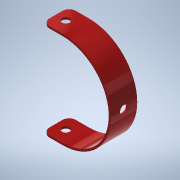
# Autodesk Inventor part: Apoio_Tubo
Saved by Autodesk Inventor 2022 (Build 260153000, 153)
## iProperties
Created: 2016-03-04
Part Number: Apoio_Tubo
Material: Genérico
Document SubType Name: Modeling
Designer: Everton
Density: 1 g/cm^3
Appearance: Padrão
Author: Everton
Autodesk Inventor part; units mm, degrees
ref_plane "YZ Plane" through (0, 0, 0) normal (1, 0, 0) x (0, 1, 0)
ref_plane "XZ Plane" through (0, 0, 0) normal (0, 1, 0) x (-1, 0, 0)
ref_plane "XY Plane" through (0, 0, 0) normal (0, 0, 1) x (1, 0, 0)
sketch "Sketch1" plane through (0, 0, 0) normal (0, 1, 0) x (-1, 0, 0)
  arc A0 (10.8783, 63.6799) -> (10.8783, -82.6701) centre (10.8783, -9.4951) ccw
  line L0 (10.8783, 63.6799) -> (40.8783, 63.6799)
  line L1 (40.8783, -82.6701) -> (10.8783, -82.6701)
  line L2 (40.8783, -79.4951) -> (10.8783, -79.4951)
  arc A1 (10.8783, 60.5049) -> (10.8783, -79.4951) centre (10.8783, -9.4951) ccw
  line L3 (10.8783, 60.5049) -> (40.8783, 60.5049)
  line L4 (40.8783, 63.6799) -> (40.8783, 60.5049)
  line L5 (40.8783, -79.4951) -> (40.8783, -82.6701)
  line L6 (25.8783, -82.6701) -> (25.8783, -9.4951)
  line L7 (25.8783, -9.4951) -> (10.8783, -9.4951)
  dimension "d1" = 30
  dimension "d2" = 3.175
  dimension "d15" = 70
  constraints: 16 end point, 4 point on circle, 2 centre point, 2 vertical, 1 collinear, 1 horizontal, 1 midpoint, 1 perpendicular, 2 other
  measures "d1" distance of L0.start L0.end
  measures "d2" radial gap between concentric circles of A0 A1
  measures "d15" radius of A1
extrude "Extrusion1" add sketch "Sketch1" along normal blind 40
sketch "Sketch2" plane through (-40.8783, 0, 63.6799) normal (0, 0, 1) x (1, 0, 0)
  line L0 (29.9701, 0) -> (0, 40)
  line L1 (0, 40) -> (30, 40)
  line L2 (0, 40) -> (30, 40) projected
  line L3 (30, 40) -> (0, 0)
  circle A0 centre (15, 20) radius 6
  point P0 (40.8783, 0)
  dimension "d5" = 12
  constraints: 6 end point, 1 centre point, 1 coincident, 1 collinear, 1 midpoint
  measures "d5" diameter of A0
extrude "Extrusion2" cut sketch "Sketch2" against normal blind 200 contours A0 L3 L0 | L0 L3 A0 | L3 A0 L0 | L0 A0 L3
fillet "Fillet1" radius 10 2 edges at (-40.8783, 40, 62.0924) (-40.8783, 0, 62.0924)
fillet "Fillet2" radius 10 2 edges at (-40.8783, 40, -81.0826) (-40.8783, 0, -81.0826)
sketch "Sketch3" plane through (-40.8783, 10, -79.4951) normal (-1, 0, 0) x (0, 0, 1)
  line L0 (-3.175, 0) -> (143.175, 20)
  line L1 (143.175, -10) -> (143.175, 30) projected
  line L2 (143.175, 0) -> (-3.175, 20)
  circle A0 centre (70, 10) radius 6
  point P0 (79.4951, -10)
  dimension "d10" = 12
  constraints: 4 end point, 2 point on line, 1 centre point, 1 midpoint
  measures "d10" diameter of A0
extrude "Extrusion3" cut sketch "Sketch3" against normal blind 200 contours A0 L2 L0 | L0 L2 A0 | L2 A0 L0 | L0 A0 L2
body "Solid1"
